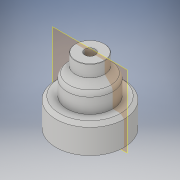
# Autodesk Inventor part: plasma tip handheld
Saved by Autodesk Inventor 2019 (Build 230136000, 136)
## iProperties
Created: 2019-01-23
Part Number: plasma tip handheld
Material: Generic
Document SubType Name: Modeling
Designer: torba
Density: 1 g/cm^3
Appearance: Default
Author: torba
Autodesk Inventor part; units mm, degrees
ref_plane "YZ Plane" through (0, 0, 0) normal (1, 0, 0) x (0, 1, 0)
ref_plane "XZ Plane" through (0, 0, 0) normal (0, 1, 0) x (-1, 0, 0)
sketch "Sketch1" plane through (0, 0, 0) normal (0, 1, 0) x (-1, 0, 0)
  circle A0 centre (0, 0) radius 12.7
  dimension "d0" = 25.4
  constraints: 1 centre point, 1 coincident
  measures "d0" diameter of A0
extrude "Extrusion1" add sketch "Sketch1" along normal blind 10.414
chamfer "Chamfer1" distance 1.27 angle 45 1 edges at (12.7, 10.414, 0)
sketch "Sketch2" plane through (0, 10.414, 0) normal (0, 1, 0) x (1, 0, 0)
  circle A0 centre (0, 0) radius 8.5344
  dimension "d6" = 17.0688
  constraints: 1 centre point, 1 coincident
  measures "d6" diameter of A0
extrude "Extrusion2" add sketch "Sketch2" along normal blind 9.6774
chamfer "Chamfer2" distance 3.048 angle 45 1 edges at (-8.5344, 20.0914, 0)
fillet "Fillet1" radius 2.54 1 edges at (-8.5344, 17.0434, 0)
sketch "Sketch3" plane through (0, 20.0914, 0) normal (0, 1, 0) x (1, 0, 0)
  circle A0 centre (0, 0) radius 5.4673
  dimension "d13" = 10.9347
  constraints: 1 centre point, 1 coincident
  measures "d13" diameter of A0
extrude "Extrusion3" add sketch "Sketch3" along normal blind 4.4704
fillet "Fillet2" radius 0.127 1 edges at (-5.4673, 24.5618, 0)
sketch "Sketch4" plane through (0, 24.5618, 0) normal (0, 1, 0) x (1, 0, 0)
  circle A0 centre (0, 0) radius 1.9685
  dimension "d17" = 3.937
  constraints: 1 centre point, 1 coincident
  measures "d17" diameter of A0
extrude "Extrusion4" cut sketch "Sketch4" against normal blind 24.638
sketch "Sketch5" plane through (0, 0, 0) normal (0, 0, 1) x (1, 0, 0)
  point P0 (0, 0)
body "Solid1"
